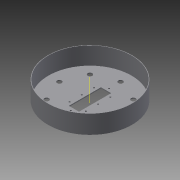
# Autodesk Inventor part: Bottom Cap
Saved by Autodesk Inventor 2015 (Build 190159000, 159)
## iProperties
Created: 2014-06-24
Part Number: Bottom Cap
Material: Generic
Document SubType Name: Modeling
Designer: Aki
Density: 1 g/cm^3
Appearance: Default
Author: Aki
Autodesk Inventor part; units mm, degrees
ref_plane "XZ Plane" through (0, 0, 0) normal (0, 1, 0) x (-1, 0, 0)
ref_plane "XY Plane" through (0, 0, 0) normal (0, 0, 1) x (1, 0, 0)
sketch "Sketch1" plane through (0, 0, 0) normal (0, 1, 0) x (-1, 0, 0)
  circle A0 centre (0, 0) radius 87
  line L0 (10.5, 33.25) -> (-10.5, 33.25)
  line L1 (-10.5, 33.25) -> (-10.5, -33.25)
  line L2 (-10.5, -33.25) -> (10.5, -33.25)
  line L3 (10.5, -33.25) -> (10.5, 33.25)
  line L4 (10.5, 33.25) -> (-10.5, -33.25) construction
  line L5 (-10.5, 33.25) -> (10.5, -33.25) construction
  circle A1 centre (16.85, 0) radius 1.5875
  circle A2 centre (-16.85, 0) radius 1.5875
  circle A3 centre (16.85, 25.4) radius 1.5875
  circle A4 centre (-16.85, 25.4) radius 1.5875
  circle A5 centre (16.85, -25.4) radius 1.5875
  circle A6 centre (-16.85, -25.4) radius 1.5875
  circle A7 centre (0, 39.6) radius 1.5875
  circle A8 centre (0, -39.6) radius 1.5875
  circle A9 centre (63.5, 0.0229) radius 4.7625
  circle A10 centre (0.0459, -63.5) radius 4.7625
  circle A11 centre (44.9256, -44.8769) radius 4.7625
  circle A12 centre (44.8932, 44.9094) radius 4.7625
  circle A13 centre (0, 63.5) radius 4.7625
  circle A14 centre (-63.5, -0.0688) radius 4.7625
  circle A15 centre (-44.8932, 44.9094) radius 4.7625
  circle A16 centre (-44.8607, -44.9418) radius 4.7625
  dimension "d0" = 174
  dimension "d1" = 21
  dimension "d2" = 66.5
  dimension "d3" = 3.175
  dimension "d4" = 3.175
  dimension "d5" = 3.175
  dimension "d6" = 3.175
  dimension "d7" = 3.175
  dimension "d8" = 3.175
  dimension "d9" = 3.175
  dimension "d10" = 3.175
  dimension "d11" = 6.35
  dimension "d13" = 0
  dimension "d14" = 0
  dimension "d15" = 6.35
  dimension "d16" = 0
  dimension "d17" = 0
  dimension "d18" = 6.35
  dimension "d19" = 6.35
  dimension "d20" = 9.525
  dimension "d21" = 9.525
  dimension "d22" = 9.525
  dimension "d23" = 9.525
  dimension "d24" = 9.525
  dimension "d25" = 9.525
  dimension "d27" = 9.525
  dimension "d28" = 9.525
  dimension "d29" = 63.5
  dimension "d30" = 63.5
  dimension "d31" = 63.5
  dimension "d32" = 63.5
  dimension "d33" = 63.5
  dimension "d34" = 63.5
  dimension "d35" = 63.5
  dimension "d36" = 63.5
  dimension "d37" = 48.5902
  dimension "d38" = 0
  dimension "d39" = 48.5902
  dimension "d41" = 48.5902
  dimension "d42" = 48.5902
  dimension "d43" = 48.5902
  dimension "d44" = 48.5902
  dimension "d45" = 48.5902
  dimension "d48" = 25.4
  dimension "d49" = 25.4
  dimension "d50" = 25.4
  dimension "d51" = 25.4
  constraints: 17 centre point, 12 end point, 2 midpoint, 2 parallel, 1 coincident, 1 horizontal, 1 perpendicular
  measures "d0" diameter of A0
  measures "d1" distance of L2.end L1.end
  measures "d2" distance of L1.end L0.end
  measures "d3" diameter of A1
  measures "d4" diameter of A2
  measures "d5" diameter of A3
  measures "d6" diameter of A4
  measures "d7" diameter of A5
  measures "d8" diameter of A6
  measures "d9" diameter of A7
  measures "d10" diameter of A8
  measures "d11" distance from line of A1.centre L3
  measures "d13" horizontal distance of A1.centre A5.centre
  measures "d14" horizontal distance of A3.centre A1.centre
  measures "d15" distance from line of A2.centre L1
  measures "d16" horizontal distance of A2.centre A6.centre
  measures "d17" horizontal distance of A4.centre A2.centre
  measures "d18" distance from line of A8.centre L2
  measures "d19" distance from line of L0 A7.centre
  measures "d20" diameter of A9
  measures "d21" diameter of A10
  measures "d22" diameter of A11
  measures "d23" diameter of A12
  measures "d24" diameter of A13
  measures "d25" diameter of A14
  measures "d27" diameter of A15
  measures "d28" diameter of A16
  measures "d29" distance of A9.centre point (0, 0)
  measures "d30" distance of point (0, 0) A11.centre
  measures "d31" distance of A10.centre A0.centre
  measures "d32" distance of A16.centre point (0, 0)
  measures "d33" distance of A0.centre A14.centre
  measures "d34" distance of A0.centre A15.centre
  measures "d35" distance of A13.centre A0.centre
  measures "d36" distance of A12.centre point (0, 0)
  measures "d37" distance of A15.centre A13.centre
  measures "d38" horizontal distance of A0.centre A13.centre
  measures "d39" distance of A12.centre A13.centre
  measures "d41" distance of A9.centre A12.centre
  measures "d42" distance of A11.centre A9.centre
  measures "d43" distance of A10.centre A11.centre
  measures "d44" distance of A16.centre A10.centre
  measures "d45" distance of A16.centre A14.centre
  measures "d48" distance of A5.centre A1.centre
  measures "d49" distance of A3.centre A1.centre
  measures "d50" distance of A4.centre A2.centre
  measures "d51" distance of A6.centre A2.centre
extrude "Extrusion1" add sketch "Sketch1" along normal blind 38.1
sketch "Sketch2" plane through (0, 38.1, 0) normal (0, 1, 0) x (1, 0, 0)
  circle A0 centre (0, 0) radius 86
  dimension "d52" = 172
  constraints: 1 centre point, 1 coincident
  measures "d52" diameter of A0
hole "Hole1" at (0, 38.1, 0) direction (0, -1, 0) diameter 172 depth 36.1
ref_plane "Work Plane1" through (0, 0, 0) normal (1, 0, 0) x (0, 1, 0)
body "Solid1"
